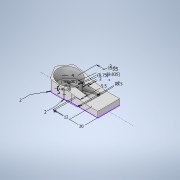
# Autodesk Inventor part: motor_arm
Saved by Autodesk Inventor 2022 (Build 260153000, 153)
## iProperties
Created: 2022-01-21
Part Number: motor_arm
Material: Generic
Document SubType Name: Modeling
Designer: felix
Density: 1 g/cm^3
Appearance: Default
Author: felix
Autodesk Inventor part; units mm, degrees
ref_plane "YZ Plane" through (0, 0, 0) normal (1, 0, 0) x (0, 1, 0)
ref_plane "XZ Plane" through (0, 0, 0) normal (0, 1, 0) x (-1, 0, 0)
ref_plane "XY Plane" through (0, 0, 0) normal (0, 0, 1) x (1, 0, 0)
sketch "Sketch1" plane through (0, 0, 0) normal (0, 1, 0) x (-1, 0, 0)
  line L0 (-1.0006, -9.2375) -> (-7.5004, -5.4843)
  line L1 (-8.5003, -3.7522) -> (-8.4997, 4.5536)
  line L2 (-8.4642, 4.9285) -> (-2.749, 8.2277)
  line L3 (8.5003, 4.5574) -> (8.4997, -3.7534)
  line L4 (7.4996, -5.4853) -> (0.9994, -9.2377)
  circle A0 centre (0, 0) radius 7.75
  circle A1 centre (0, 0) radius 2.75
  line L5 (0, 0) -> (2.8284, -2.8284)
  line L6 (0, 0) -> (4, 0) construction
  circle A2 centre (2.8284, -2.8284) radius 1
  circle A3 centre (0, 0) radius 1
  circle A4 centre (2.8284, 2.8284) radius 1
  circle A5 centre (-2.8284, 2.8284) radius 1
  circle A6 centre (-2.8284, -2.8284) radius 1
  line L7 (0.001, -18) -> (0.001, 46) construction
  line L8 (7.751, 9.815) -> (7.751, 28.2268)
  line L9 (-7.749, 9.815) -> (-7.749, 28.2268)
  arc A7 (7.4996, -5.4853) -> (8.4997, -3.7534) centre (6.4997, -3.7532) ccw
  arc A8 (-1.0006, -9.2375) -> (0.9994, -9.2377) centre (-0.0005, -7.5056) ccw
  arc A9 (-8.5003, -3.7522) -> (-7.5004, -5.4843) centre (-6.5003, -3.7523) ccw
  arc A10 (7.751, 9.815) -> (8.3891, 5.2152) centre (19.5793, 9.1116) ccw
  arc A11 (8.5003, 4.5574) -> (8.3891, 5.2152) centre (6.5003, 4.5575) ccw
  arc A12 (-8.3883, 5.2117) -> (-7.749, 9.815) centre (-19.5772, 9.1116) ccw
  arc A13 (-8.3883, 5.2117) -> (-8.4997, 4.5536) centre (-6.4997, 4.5535) ccw
  line L10 (2.751, 7.2453) -> (2.751, 8.182)
  line L11 (-2.749, 7.2453) -> (-2.749, 8.182)
  line L12 (2.751, 8.182) -> (2.751, 19.2453)
  line L13 (-2.749, 8.182) -> (-2.749, 19.2453)
  line L14 (0.0007, 9.815) -> (0.001, 9.8148)
  line L15 (2.751, 8.2268) -> (8.4659, 4.9268)
  line L16 (-7.749, 28.2268) -> (7.751, 28.2268)
  line L17 (-2.749, 19.2453) -> (2.751, 19.2453)
  line L18 (-2.749, 19.2453) -> (-7.749, 19.2453)
  line L19 (2.751, 19.2453) -> (7.751, 19.2453)
  line L20 (2.751, 19.2453) -> (2.751, 28.2268)
  line L21 (-2.749, 19.2453) -> (-2.749, 28.2268)
  point P0 (-0.0007, -9.815)
  point P1 (-8.5003, -4.9069)
  point P2 (8.4997, -4.9081)
  point P3 (-2.749, 7.2461)
  dimension "d1" = 15.5
  dimension "d0" = 17
  dimension "d2" = 0.75
  dimension "d3" = 5.5
  dimension "d4" = 4
  dimension "d5" = 45
  dimension "d6" = 2
  dimension "d7" = 2
  dimension "d10" = 360
  dimension "d12" = 9.8355
  dimension "d13" = 2
  dimension "d14" = 2
  dimension "d15" = 2
  dimension "d16" = 15.5
  dimension "d17" = 5.5
  dimension "d19" = 12
  dimension "d21" = 20
  constraints: 44 end point, 16 point on circle, 13 centre point, 12 point on line, 10 tangent, 7 coincident, 7 symmetric about line, 4 perpendicular, 4 vertical, 2 equal radius, 2 horizontal, 1 equal length, 22 other
  measures "d0" distance between parallel lines of L1 L3
  measures "d3" diameter of A1
  measures "d4" distance of L5.start L5.end
  measures "d5" angle of L5 L6
  measures "d6" diameter of A2
  measures "d7" diameter of A3
  measures "d12" distance of L2.start point (-8.5, -4.907)
  measures "d13" radius of A7
  measures "d14" radius of A11
  measures "d15" radius of A13
  measures "d16" distance between parallel lines of L9 L8
  measures "d17" distance between parallel lines of L11 L10
  measures "d19" distance of L12.end L10.start
  measures "d21" vertical distance of L8.end L15.start
extrude "Extrusion1" add sketch "Sketch1" along normal blind 0.2 contours A1
extrude "Extrusion2" add sketch "Sketch1" along normal blind 1 contours A0
extrude "Extrusion5" add sketch "Sketch1" along normal blind 1 contours L13 L17 L12 L10 A0 L11
extrude "Extrusion10" add sketch "Sketch1" along normal blind 4 contours L18 L9 L16 L21 | L20 L16 L8 L19
extrude "Extrusion11" add sketch "Sketch1" along normal blind 4 contours L21 L16 L20 L17
extrude "Extrusion12" cut sketch "Sketch1" along normal blind 4 contours L13 L17 L12 L10 A0 L11
extrude "Extrusion13" add sketch "Sketch1" along normal blind 4 contours L13 L17 L12 L10 A0 L11
extrude "Extrusion14" add sketch "Sketch1" along normal blind 8 contours L0 A9 L1 A13 L2 L13 L11 A0 L10 L12 L15 A11 L3 A7 L4 A8
ref_plane "Work Plane2" through (7.749, 4, 19.2453) normal (0, 0.9862856, 0.1650476) x (-1, 0, 0)
extrude "Extrusion15" cut sketch "Sketch1" along normal blind 8 contours L0 A9 L1 A13 L2 L13 L11 A0 L10 L12 L15 A11 L3 A7 L4 A8
extrude "Extrusion16" add sketch "Sketch1" along normal up to surface contours L0 A9 L1 A13 L2 L13 L11 A0 L10 L12 L15 A11 L3 A7 L4 A8 | A13 A12 L9 L18 L13 L2 | L15 L12 L19 L8 A10 A11 surface through (7.749, 4, 19.2453) normal (0, 0.9862856, 0.1650476)
ref_plane "Work Plane3" through (2.749, 4, 19.2453) normal (0, 0.9711343, -0.2385335) x (-1, 0, 0)
extrude "Extrusion17" cut sketch "Sketch1" along normal blind 10 contours L13 L17 L12 L10 A0 L11
extrude "Extrusion18" add sketch "Sketch1" against normal up to surface contours L13 L17 L12 L10 A0 L11 surface through (2.749, 4, 19.2453) normal (0, 0.9711343, -0.2385335)
body "Solid1"
